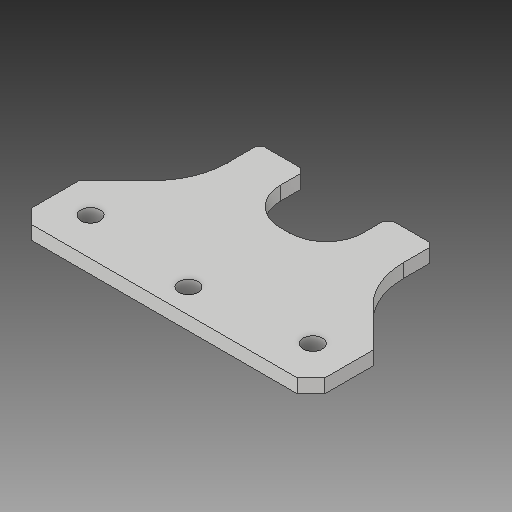
# Autodesk Inventor part: stopperver2_2
Saved by Autodesk Inventor 2018 (Build 220112000, 112)
## iProperties
Created: 2020-08-12
Part Number: stopperver2_2
Material: 一般
Document SubType Name: Modeling
Designer: gisen
Density: 1 g/cm^3
Appearance: 既定
Mass: 5.34888 g
Surface Area: 43.0168 cm^2
Volume: 5.34888 cm^3
Author: gisen
Autodesk Inventor part; units mm, degrees
ref_plane "YZ Plane" through (0, 0, 0) normal (1, 0, 0) x (0, 1, 0)
ref_plane "XZ Plane" through (0, 0, 0) normal (0, 1, 0) x (-1, 0, 0)
ref_plane "XY Plane" through (0, 0, 0) normal (0, 0, 1) x (1, 0, 0)
sketch "スケッチ3" plane through (0, 0, 0) normal (0, 1, 0) x (-1, 0, 0)
  circle A0 centre (55.3, 11.85) radius 2.1
  circle A1 centre (31.1, 14.7) radius 2.1
  circle A2 centre (6.9, 11.85) radius 2.1
  line L0 (62.1, 5.5) -> (0.1, 5.5)
  line L1 (2.1, 20) -> (60.1, 20)
  line L2 (-0.9, 6.5) -> (-0.9, 17)
  line L3 (63.1, 17) -> (63.1, 6.5)
  line L4 (49.3, -20) -> (41.3, -20)
  line L5 (21.3, -20) -> (13.3, -20)
  line L6 (63.1, 17) -> (60.1, 20)
  line L7 (2.1, 20) -> (-0.9, 17)
  line L8 (50.3, -19) -> (50.3, 5.5)
  line L9 (40.3, -19) -> (40.3, 5.5)
  line L10 (22.3, -19) -> (22.3, 5.5)
  line L11 (12.3, -19) -> (12.3, 5.5)
  line L12 (62.1, 5.5) -> (63.1, 6.5)
  line L13 (0.1, 5.5) -> (-0.9, 6.5)
  line L14 (12.3, -19) -> (13.3, -20)
  line L15 (22.3, -19) -> (21.3, -20)
  line L16 (40.3, -19) -> (41.3, -20)
  line L17 (50.3, -19) -> (49.3, -20)
  point P0 (0, 0)
  point P1 (-0.9, 20)
  point P2 (-0.9, 5.5)
  point P3 (63.1, 5.5)
  point P4 (50.3, -20)
  point P5 (40.3, -20)
  point P6 (22.3, -20)
  point P7 (12.3, -20)
  point P8 (61.6, 18.5)
  dimension "d2" = 3
  dimension "d3" = 3
  dimension "d4" = 4.2
  dimension "d5" = 4.2
  dimension "d6" = 4.2
  dimension "d7" = 10
  dimension "d8" = 10
  dimension "d11" = 1
  dimension "d12" = 1
  dimension "d13" = 1
  dimension "d14" = 1
  dimension "d16" = 1
  dimension "d17" = 1
  dimension "d18" = 1
  dimension "d19" = 1
  dimension "d20" = 1
  dimension "d21" = 1
  dimension "d22" = 1
  constraints: 36 end point, 17 point on line, 5 vertical, 3 centre point, 3 perpendicular, 2 horizontal, 1 midpoint, 4 other
  measures "d2" distance of L1.start point (-0.9, 20)
  measures "d3" distance of L2.end point (-0.9, 20)
  measures "d4" diameter of A0
  measures "d5" diameter of A1
  measures "d6" diameter of A2
  measures "d7" distance between parallel lines of L8 L9
  measures "d8" distance between parallel lines of L11 L10
  measures "d11" distance of L0.start point (63.1, 5.5)
  measures "d12" distance of L3.end point (63.1, 5.5)
  measures "d13" distance of L0.end point (-0.9, 5.5)
  measures "d14" distance of L2.start point (-0.9, 5.5)
  measures "d16" distance of L5.end point (12.3, -20)
  measures "d17" distance of L10.start point (22.3, -20)
  measures "d18" distance of L5.start point (22.3, -20)
  measures "d19" distance of L9.start point (40.3, -20)
  measures "d20" distance of L4.end point (40.3, -20)
  measures "d21" distance of L8.start point (50.3, -20)
  measures "d22" distance of L4.start point (50.3, -20)
extrude "押し出し1" add sketch "スケッチ3" along normal blind 3
sketch "スケッチ4" plane through (0, 0, 0) normal (0, -1, 0) x (1, 0, 0)
  line L0 (-40.3, 5.5) -> (-22.3, 5.5)
  line L1 (-22.3, 5.5) -> (-22.3, -6.5)
  line L2 (-22.3, -6.5) -> (-40.3, -6.5)
  line L3 (-40.3, -6.5) -> (-40.3, 5.5)
  line L4 (-22.3, -19) -> (-22.3, 5.5) projected
  point P0 (0, 0)
  dimension "d23" = 12
  constraints: 8 end point, 2 parallel, 1 horizontal, 1 perpendicular, 1 point on line
  measures "d23" distance between parallel lines of L0 L2
extrude "押し出し2" add sketch "スケッチ4" against normal blind 3
sketch "スケッチ5" plane through (0, 0, 0) normal (0, -1, 0) x (1, 0, 0)
  line L0 (-0.1, 5.5) -> (-12.3, 5.5)
  line L1 (-12.3, 5.5) -> (-12.3, -6.7)
  line L2 (-12.3, -6.7) -> (-0.1, 5.5)
  line L3 (0.9, 6.5) -> (-0.1, 5.5) projected
  line L4 (-50.3, -6.3) -> (-50.3, 5.5)
  line L5 (-50.3, 5.5) -> (-62.1, 5.5)
  line L6 (-62.1, 5.5) -> (-50.3, -6.3)
  line L7 (-62.1, 5.5) -> (-63.1, 6.5) projected
  point P0 (0, 0)
  constraints: 12 end point, 4 coincident, 2 collinear, 2 perpendicular, 1 horizontal, 1 vertical
extrude "押し出し3" add sketch "スケッチ5" against normal blind 3
fillet "フィレット2" radius 8 2 edges at (-22.3, 1.5, -6.5) (-40.3, 1.5, -6.5)
fillet "フィレット2" radius 16 2 edges at (-12.3, 1.5, -6.7) (-50.3, 1.5, -6.3)
equation "\"d2\" = d0"
equation "\"d3\" = d2"
equation "\"d7\" = d8"
equation "\"d12\" = d11"
equation "\"d13\" = d11"
equation "\"d14\" = d13"
equation "\"d16\" = d15"
equation "\"d17\" = d11"
equation "\"d18\" = d17"
equation "\"d19\" = d11"
equation "\"d20\" = d19"
equation "\"d21\" = d11"
equation "\"d22\" = d21"
equation "\"d15\" = d11"
equation "\"d0\" = 3"
